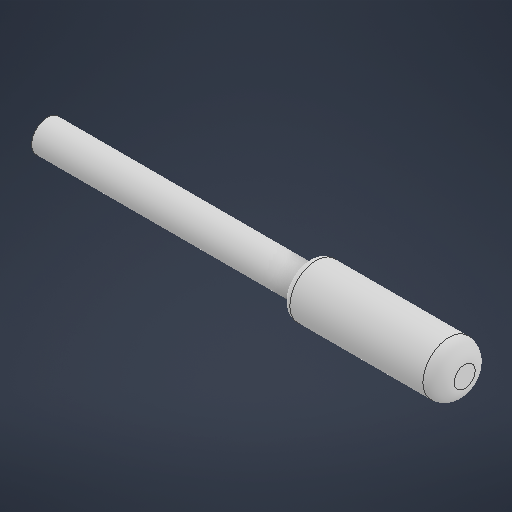
# Autodesk Inventor part: součást 3
Saved by Autodesk Inventor 2025.1 (Build 291241000, 241)
## iProperties
Created: 2025-04-28
Part Number: součást 3
Material: Všeobecné
Document SubType Name: Modeling
Designer: Dominik Petříček
Density: 1 g/cm^3
Appearance: Výchozí
Author: Dominik Petříček
Autodesk Inventor part; units mm, degrees
ref_plane "YZ Plane" through (0, 0, 0) normal (1, 0, 0) x (0, 1, 0)
ref_plane "XZ Plane" through (0, 0, 0) normal (0, 1, 0) x (-1, 0, 0)
ref_plane "XY Plane" through (0, 0, 0) normal (0, 0, 1) x (1, 0, 0)
sketch "Náčrt1" plane through (0, 0, 0) normal (0, 0, 1) x (1, 0, 0)
  line L0 (0, 0) -> (0, -3)
  line L1 (0, -3) -> (50, -3)
  line L2 (50, -3) -> (50, 0)
  line L3 (50, 0) -> (80, 0)
  line L4 (80, 0) -> (80, -2)
  line L5 (77, -5) -> (51.5, -5)
  line L6 (50, -3.5) -> (50, -3)
  arc A0 (50, -3.5) -> (51.5, -5) centre (51.5, -3.5) ccw
  arc A1 (77, -5) -> (80, -2) centre (77, -2) ccw
  line L7 (50, 0) -> (0, 0)
  point P0 (80, -5)
  point P1 (50, -5)
  dimension "d0" = 3
  dimension "d1" = 50
  dimension "d2" = 30
  dimension "d3" = 5
  dimension "d4" = 1.5
  dimension "d5" = 3
  constraints: 16 end point, 6 perpendicular, 5 point on line, 4 point on circle, 4 tangent, 2 centre point, 1 horizontal, 1 vertical
  measures "d0" distance of L0.start L0.end
  measures "d1" distance of L0.end L1.end
  measures "d2" distance of L2.end L3.end
  measures "d3" distance of L3.end point (80, -5)
  measures "d4" radius of A0
  measures "d5" radius of A1
revolve "Rotace1" add sketch "Náčrt1" angle 360 about axis through (50, 0, 0) along (-1, 0, 0)
